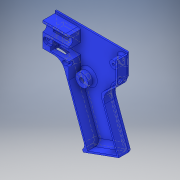
# Autodesk Inventor part: Griff_rechts
Saved by Autodesk Inventor 2019 (Build 230136000, 136)
## iProperties
Created: 2021-03-07
Part Number: Griff_rechts
Material: Generic
Document SubType Name: Modeling
Designer: Lukas
Density: 1 g/cm^3
Appearance: Default
Author: Lukas
Autodesk Inventor part; units mm, degrees
ref_plane "YZ Plane" through (0, 0, 0) normal (1, 0, 0) x (0, 1, 0)
ref_plane "XZ Plane" through (0, 0, 0) normal (0, 1, 0) x (-1, 0, 0)
ref_plane "XY Plane" through (0, 0, 0) normal (0, 0, 1) x (1, 0, 0)
sketch "Sketch1" plane through (0, 0, 0) normal (0, 0, 1) x (1, 0, 0)
  line L0 (-51.5891, 42.2862) -> (-20.8072, -42.2862)
  line L1 (-20.8072, -42.2862) -> (-24.5184, -46.7089)
  line L2 (-24.5184, -46.7089) -> (-23.4923, -49.528)
  line L3 (-23.4923, -49.528) -> (23.4923, -32.427)
  line L4 (21.261, 47.2862) -> (1.261, 28.653)
  line L5 (1.261, 28.653) -> (23.4923, -32.427)
  line L6 (0, -74.8908) -> (0, 102.649) projected
  line L7 (-76.5891, 77.2862) -> (21.261, 77.2862)
  line L8 (21.261, 77.2862) -> (21.261, 47.2862)
  line L9 (-51.5891, 42.2862) -> (-76.5891, 42.2862)
  line L10 (-76.5891, 42.2862) -> (-76.5891, 77.2862)
  point P0 (0, 0)
  point P1 (-36.1981, 0)
  point P2 (0, -40.9775)
  dimension "d1" = 90
  dimension "d2" = 120
  dimension "d3" = 3
  dimension "d5" = 45
  dimension "d6" = 20
  dimension "d7" = 65
  dimension "d8" = 5
  dimension "d10" = 30
  dimension "d30" = 20
  dimension "d31" = 25
  dimension "d32" = 35
  constraints: 21 end point, 5 perpendicular, 2 midpoint, 1 horizontal, 1 horizontal alignment, 1 parallel, 1 vertical alignment
  measures "d1" distance of L0.start L0.end
  measures "d2" angle of L0 L1
  measures "d3" distance of L1.end L2.end
  measures "d5" distance between parallel lines of L5 L0
  measures "d6" angle of L6 L0
  measures "d7" distance of L4.end L3.end
  measures "d8" distance between parallel lines of L2 L0
  measures "d10" distance of L7.end L4.start
  measures "d30" distance from line of L8 L4.end
  measures "d31" distance of L0.start L9.end
  measures "d32" distance of L9.end L7.start
extrude "Extrusion1" add sketch "Sketch1" along normal blind 2
sketch "Sketch2" plane through (0, 0, 2) normal (0, 0, 1) x (1, 0, 0)
  line L0 (-51.5891, 42.2862) -> (-20.8072, -42.2862) projected
  line L1 (-20.8072, -42.2862) -> (-24.5184, -46.7089) projected
  line L2 (-24.5184, -46.7089) -> (-23.4923, -49.528) projected
  line L3 (-23.4923, -49.528) -> (23.4923, -32.427) projected
  line L4 (23.4923, -32.427) -> (1.261, 28.653) projected
  line L5 (1.261, 28.653) -> (21.261, 47.2862) projected
  line L6 (21.261, 47.2862) -> (21.261, 77.2862) projected
  line L7 (21.261, 77.2862) -> (-76.5891, 77.2862) projected
  circle A0 centre (-32.3938, 24.6332) radius 3
  circle A1 centre (-32.3938, 24.6332) radius 8.5
  line L8 (-76.5891, 77.2862) -> (-76.5891, 42.2862) projected
  line L9 (-76.5891, 42.2862) -> (-51.5891, 42.2862) projected
  point P0 (0, 0)
  dimension "d14" = 20
  dimension "d15" = 33
  dimension "d55" = 6
  dimension "d56" = 17
  constraints: 2 centre point, 1 coincident
  measures "d14" distance from line of L5 A0.centre
  measures "d15" distance from line of L4 A0.centre
  measures "d55" diameter of A0
  measures "d56" diameter of A1
extrude "Extrusion2" add sketch "Sketch2" along normal blind 9 contours A1
sketch "Sketch3" plane through (0, 0, 2) normal (0, 0, 1) x (1, 0, 0)
  line L0 (-51.5891, 42.2862) -> (-20.8072, -42.2862) projected
  line L1 (-20.8072, -42.2862) -> (-24.5184, -46.7089) projected
  line L2 (-24.5184, -46.7089) -> (-23.4923, -49.528) projected
  line L3 (-23.4923, -49.528) -> (23.4923, -32.427) projected
  line L4 (23.4923, -32.427) -> (1.261, 28.653) projected
  line L5 (1.261, 28.653) -> (21.261, 47.2862) projected
  line L6 (21.261, 47.2862) -> (21.261, 77.2862) projected
  line L7 (21.261, 77.2862) -> (-76.5891, 77.2862) projected
  circle A0 centre (-32.3938, 24.6332) radius 8.5 projected
  line L8 (-50.1886, 44.2862) -> (-17.5985, -45.2545)
  line L9 (-17.5985, -45.2545) -> (20.9289, -31.2317)
  line L10 (20.9289, -31.2317) -> (-1.0714, 29.2135)
  line L11 (-1.0714, 29.2135) -> (19.261, 48.1563)
  line L12 (19.261, 48.1563) -> (19.261, 77.2862)
  line L13 (21.261, 77.2862) -> (-76.5891, 77.2862) projected
  line L14 (1.261, 28.653) -> (21.261, 47.2862) projected
  line L15 (23.4923, -32.427) -> (1.261, 28.653) projected
  line L16 (-51.5891, 42.2862) -> (-20.8072, -42.2862) projected
  line L17 (-24.5184, -46.7089) -> (-20.8072, -42.2862) projected
  line L18 (-51.5891, 42.2862) -> (-20.8072, -42.2862)
  line L19 (-20.8072, -42.2862) -> (-24.5184, -46.7089)
  line L20 (-24.5184, -46.7089) -> (-23.4923, -49.528)
  line L21 (23.4923, -32.427) -> (-23.4923, -49.528)
  line L22 (-23.4923, -49.528) -> (23.4923, -32.427) projected
  line L23 (23.4923, -32.427) -> (1.261, 28.653)
  line L24 (1.261, 28.653) -> (21.261, 47.2862)
  line L25 (21.261, 77.2862) -> (21.261, 47.2862)
  line L26 (19.261, 77.2862) -> (21.261, 77.2862)
  line L27 (-76.5891, 77.2862) -> (-76.5891, 42.2862) projected
  line L28 (-76.5891, 42.2862) -> (-51.5891, 42.2862) projected
  line L29 (-76.5891, 77.2862) -> (-76.5891, 42.2862) projected
  line L30 (-51.5891, 42.2862) -> (-76.5891, 42.2862)
  line L31 (-76.5891, 42.2862) -> (-76.5891, 44.2862)
  line L32 (-76.5891, 44.2862) -> (-50.1886, 44.2862)
  point P0 (-51.5891, 77.2862)
  dimension "d20" = 2
  dimension "d21" = 2
  dimension "d22" = 2
  dimension "d23" = 2
  dimension "d24" = 2
  dimension "d33" = 2
  constraints: 32 end point, 6 perpendicular, 5 parallel, 2 point on line, 2 vertical, 1 collinear, 1 horizontal
  measures "d20" distance between parallel lines of L6 L12
  measures "d21" distance between parallel lines of L16 L8
  measures "d22" distance between parallel lines of L4 L10
  measures "d23" distance between parallel lines of L14 L11
  measures "d24" distance between parallel lines of L3 L9
  measures "d33" distance between parallel lines of L32 L28
extrude "Extrusion3" add sketch "Sketch3" along normal blind 16 contours L28 L27 L32 L8 L9 L10 L11 L12 L7 L6 L5 L4 L3 L2 L1 L0
fillet "Fillet1" radius 6 2 edges at (9.9288, -1.0091, 2) (1.6652, -38.2431, 2)
fillet "Fillet3" radius 15 2 edges at (1.261, 28.653, 9) (-51.5891, 42.2862, 9)
fillet "Fillet2" radius 8 3 edges at (21.261, 47.2862, 9) (-20.8072, -42.2862, 9) (-1.0714, 29.2135, 13)
sketch "Sketch4" plane through (0, 0, 2) normal (0, 0, 1) x (1, 0, 0)
  line L0 (-76.5891, 77.2862) -> (-76.5891, 44.2862) projected
  line L1 (-76.5891, 74.2862) -> (-42.3941, 74.2862)
  line L2 (-42.3941, 74.2862) -> (-42.3941, 58.2862)
  line L3 (-42.3941, 58.2862) -> (-76.5891, 58.2862)
  line L4 (-76.5891, 58.2862) -> (-76.5891, 74.2862)
  line L5 (19.261, 77.2862) -> (-76.5891, 77.2862) projected
  line L6 (-50.1886, 44.2862) -> (-76.5891, 44.2862) projected
  point P0 (0, 0)
  point P1 (11.261, 77.2862)
  point P2 (-76.5891, 52.2862)
  point P3 (-59.2913, 46.2862)
  dimension "d34" = 34.195
  dimension "d35" = 3
  dimension "d42" = 14
  constraints: 8 end point, 2 parallel, 1 horizontal, 1 perpendicular, 1 point on line, 1 other
  measures "d34" distance of L1.start L1.end
  measures "d35" distance between parallel lines of L5 L1
extrude "Extrusion4" add sketch "Sketch4" along normal blind 16
sketch "Sketch5" plane through (-76.5891, 77.2862, 0) normal (-1, 0, 0) x (0, 0, 1)
  line L0 (18, -3) -> (18, -19) projected
  circle A0 centre (18, -11) radius 5
  point P0 (0, -77.2862)
  dimension "d39" = 10
  constraints: 1 centre point, 1 midpoint
  measures "d39" diameter of A0
extrude "Extrusion5" cut sketch "Sketch5" against normal up to surface (34.195 mm away)
sketch "Sketch6" plane through (0, 0, 2) normal (0, 0, 1) x (1, 0, 0)
  line L0 (-42.3941, 58.2862) -> (-76.5891, 58.2862) projected
  line L1 (-76.5891, 58.2862) -> (-76.5891, 44.2862)
  line L2 (-66.5891, 44.2862) -> (-66.5891, 58.2862)
  line L3 (-76.5891, 58.2862) -> (-66.5891, 58.2862)
  line L4 (-66.5891, 44.2862) -> (-76.5891, 44.2862)
  point P0 (0, 0)
  dimension "d53" = 10
  constraints: 8 end point, 1 coincident, 1 collinear, 1 horizontal, 1 parallel, 1 perpendicular
  measures "d53" distance between parallel lines of L1 L2
extrude "Extrusion6" add sketch "Sketch6" along normal blind 16
sketch "Sketch7" plane through (0, 0, 18) normal (0, 0, 1) x (1, 0, 0)
  circle A0 centre (-72.0891, 53.2862) radius 4
  circle A1 centre (-72.0891, 53.2862) radius 1.45
  line L0 (-72.0891, 57.2862) -> (-66.5891, 57.2862)
  line L1 (-72.0891, 49.2862) -> (-66.5891, 49.2862)
  line L2 (-66.5891, 44.2862) -> (-66.5891, 58.2862) projected
  line L3 (-66.5891, 58.2862) -> (-42.3941, 58.2862) projected
  point P0 (0, 0)
  point P1 (-66.5891, 51.2862)
  dimension "d47" = 2.9
  dimension "d48" = 8
  dimension "d54" = 5.5
  dimension "d66" = 5
  constraints: 4 end point, 2 centre point, 2 horizontal, 2 point on circle, 2 point on line, 2 tangent, 1 coincident, 1 midpoint
  measures "d47" diameter of A1
  measures "d48" diameter of A0
  measures "d54" distance from line of L2 A0.centre
  measures "d66" distance from line of A0.centre L3
extrude "Extrusion7" cut sketch "Sketch7" against normal blind 3
extrude "Extrusion8" cut sketch "Sketch7" against normal blind 15 contours A1
sketch "Sketch8" plane through (0, 0, 2) normal (0, 0, 1) x (1, 0, 0)
  line L0 (-22.387, -37.9459) -> (-51.5891, 42.2862) projected
  line L1 (-17.5985, -45.2545) -> (-50.1886, 44.2862) projected
  line L2 (-76.5891, 42.2862) -> (-62.0922, 42.2862) projected
  line L3 (-50.1886, 44.2862) -> (-66.5891, 44.2862) projected
  line L4 (-42.3941, 58.2862) -> (-66.5891, 58.2862) projected
  line L5 (-66.5891, 58.2862) -> (-42.3941, 58.2862) projected
  line L6 (-42.3941, 71.2862) -> (-42.3941, 61.2862) projected
  line L7 (-42.3941, 71.2862) -> (-42.3941, 74.2862) projected
  line L8 (-42.3941, 74.2862) -> (-42.3941, 58.2862) projected
  circle A0 centre (-32.3938, 24.6332) radius 8.5 projected
  circle A1 centre (-32.3938, 24.6332) radius 8.5 projected
  line L9 (-50.1886, 44.2862) -> (-42.3941, 44.2862)
  line L10 (-42.3941, 44.2862) -> (-42.3941, 22.8707)
  line L11 (-42.3941, 22.8707) -> (-50.1886, 44.2862)
  line L12 (-42.3941, 58.2862) -> (-42.3941, 61.2862) projected
  line L13 (-66.5891, 44.2862) -> (-50.1886, 44.2862) projected
  line L14 (-17.5985, -45.2545) -> (-19.6506, -39.6163) projected
  line L15 (-50.1886, 44.2862) -> (-19.6506, -39.6163) projected
  line L16 (-66.5891, 44.2862) -> (-50.1886, 44.2862) projected
  line L17 (-62.0922, 42.2862) -> (-76.5891, 42.2862) projected
  point P0 (0, 0)
  point P1 (-48.7882, 46.2862)
  point P2 (-48.7882, 46.2862)
  point P3 (-48.7882, 46.2862)
  constraints: 6 end point, 2 collinear, 2 horizontal, 1 perpendicular, 1 point on line, 1 other
extrude "Extrusion9" add sketch "Sketch8" along normal blind 16 contours L1 L9 L10
sketch "Sketch9" plane through (0, 0, 18) normal (0, 0, 1) x (1, 0, 0)
  circle A0 centre (-47.6301, 40.2862) radius 3
  line L0 (-45.3941, 42.2862) -> (-42.3941, 42.2862)
  line L1 (-42.3941, 44.2862) -> (-42.3941, 22.8707) projected
  line L2 (-45.3941, 38.2862) -> (-42.3941, 38.2862)
  line L3 (-42.3941, 22.8707) -> (-42.3941, 44.2862) projected
  line L4 (-42.3941, 44.2862) -> (-66.5891, 44.2862) projected
  point P0 (0, 0)
  point P1 (-66.5891, 44.2862)
  point P2 (-59.2913, 46.2862)
  dimension "d60" = 6
  dimension "d61" = 4
  dimension "d62" = 3
  dimension "d63" = 4
  constraints: 4 end point, 2 point on circle, 2 point on line, 1 centre point, 1 horizontal, 1 perpendicular, 1 vertical alignment, 1 other
  measures "d60" diameter of A0
  measures "d61" distance between parallel lines of L2 L0
  measures "d62" distance of L0.start L0.end
extrude "Extrusion10" cut sketch "Sketch9" against normal blind 5
sketch "Sketch10" plane through (0, 0, 18) normal (0, 0, 1) x (1, 0, 0)
  line L0 (-76.5891, 71.2862) -> (-42.3941, 71.2862) projected
  line L1 (-42.3941, 61.2862) -> (-76.5891, 61.2862) projected
  line L2 (-76.5891, 61.2862) -> (-76.5891, 71.2862) projected
  line L3 (-76.5891, 74.2862) -> (-76.5891, 71.2862) projected
  line L4 (-76.5891, 77.2862) -> (-76.5891, 74.2862) projected
  line L5 (-76.5891, 42.2862) -> (-76.5891, 77.2862) projected
  line L6 (-76.5891, 61.2862) -> (-76.5891, 42.2862) projected
  line L7 (-42.3941, 71.2862) -> (-42.3941, 61.2862) projected
  line L8 (-42.3941, 58.2862) -> (-42.3941, 61.2862) projected
  line L9 (-42.3941, 74.2862) -> (-42.3941, 58.2862) projected
  line L10 (-42.3941, 71.2862) -> (-42.3941, 74.2862) projected
  line L11 (-67.3941, 68.5362) -> (-47.3941, 68.5362)
  line L12 (-47.3941, 68.5362) -> (-47.3941, 64.0362)
  line L13 (-47.3941, 64.0362) -> (-67.3941, 64.0362)
  line L14 (-67.3941, 64.0362) -> (-67.3941, 68.5362)
  point P0 (0, 0)
  dimension "d67" = 2.75
  dimension "d68" = 2.75
  dimension "d69" = 4.5
  dimension "d70" = 5
  dimension "d71" = 20
  constraints: 8 end point, 2 parallel, 1 horizontal, 1 perpendicular
  measures "d67" distance between parallel lines of L0 L11
  measures "d68" distance between parallel lines of L1 L13
  measures "d69" distance of L13.end L11.start
  measures "d70" distance between parallel lines of L7 L12
  measures "d71" distance of L11.start L11.end
extrude "Extrusion11" cut sketch "Sketch10" against normal through all contours L11 L12 L13 L14
sketch "Sketch11" plane through (0, 0, 2) normal (0, 0, 1) x (1, 0, 0)
  circle A0 centre (13.261, 67.2862) radius 5
  line L0 (19.261, 77.2862) -> (19.261, 48.1563) projected
  line L1 (19.261, 48.1563) -> (2.8048, 32.8248) projected
  line L2 (8.5288, 35.4241) -> (18.7143, 44.9135) projected
  arc A1 (18.7143, 44.9135) -> (21.261, 50.7669) centre (13.261, 50.7669) ccw projected
  line L3 (21.261, 50.7669) -> (21.261, 77.2862) projected
  line L4 (-76.5891, 77.2862) -> (21.261, 77.2862) projected
  line L5 (19.261, 77.2862) -> (-76.5891, 77.2862) projected
  line L6 (21.261, 77.2862) -> (19.261, 77.2862) projected
  line L7 (0.4724, 33.3853) -> (17.261, 49.0265) projected
  circle A2 centre (13.261, 67.2862) radius 1.45
  line L8 (21.261, 77.2862) -> (21.261, 50.7669) projected
  arc A3 (18.7143, 44.9135) -> (21.261, 50.7669) centre (13.261, 50.7669) ccw projected
  line L9 (18.7143, 44.9135) -> (8.5288, 35.4241) projected
  line L10 (2.8048, 32.8248) -> (1.7313, 31.8246) projected
  line L11 (1.7313, 31.8246) -> (19.261, 48.1563) projected
  line L12 (19.261, 48.1563) -> (19.261, 77.2862) projected
  point P0 (0, 0)
  dimension "d75" = 10
  dimension "d76" = 10
  dimension "d77" = 2.9
  dimension "d121" = 6
  constraints: 2 centre point, 1 coincident
  measures "d75" distance from line of L4 A0.centre
  measures "d76" diameter of A0
  measures "d77" diameter of A2
  measures "d121" distance from line of L0 A0.centre
extrude "Extrusion12" add sketch "Sketch11" along normal blind 13
sketch "Sketch17" plane through (0, 0, 2) normal (0, 0, 1) x (1, 0, 0)
  circle A0 centre (-59.5891, 54.2862) radius 4
  circle A1 centre (-59.5891, 54.2862) radius 1.45
  line L0 (-42.3941, 58.2862) -> (-66.5891, 58.2862) projected
  line L1 (-66.5891, 58.2862) -> (-42.3941, 58.2862) projected
  line L2 (-66.5891, 57.2862) -> (-66.5891, 49.2862) projected
  line L3 (-66.5891, 44.2862) -> (-66.5891, 49.2862) projected
  line L4 (-66.5891, 58.2862) -> (-66.5891, 44.2862) projected
  line L5 (-66.5891, 57.2862) -> (-66.5891, 58.2862) projected
  line L6 (-42.3941, 71.2862) -> (-42.3941, 61.2862) projected
  line L7 (-42.3941, 71.2862) -> (-42.3941, 74.2862) projected
  line L8 (-42.3941, 74.2862) -> (-42.3941, 58.2862) projected
  line L9 (-42.3941, 58.2862) -> (-42.3941, 61.2862) projected
  point P0 (0, 0)
  dimension "d109" = 2.9
  dimension "d110" = 8
  dimension "d111" = 4
  dimension "d112" = 7
  constraints: 2 centre point, 1 coincident
  measures "d109" diameter of A1
  measures "d110" diameter of A0
  measures "d111" distance from line of L0 A0.centre
  measures "d112" distance from line of L2 A0.centre
extrude "Extrusion18" add sketch "Sketch17" along normal blind 3
sketch "Sketch12" plane through (19.261, 48.1563, 18) normal (-1, 0, 0) x (0, 0, 1)
  circle A0 centre (-4, 4) radius 3.5
  line L0 (0, 29.1298) -> (0, 0) projected
  line L1 (-16, 0) -> (0, 0) projected
  point P0 (-18, -48.1563)
  point P1 (-10, 0)
  dimension "d81" = 4
  dimension "d82" = 7
  dimension "d83" = 4
  constraints: 1 centre point
  measures "d81" distance from line of L0 A0.centre
  measures "d82" diameter of A0
  measures "d83" distance from line of L1 A0.centre
extrude "Extrusion13" cut sketch "Sketch12" against normal blind 2
sketch "Sketch14" plane through (-76.5891, 42.2862, 18) normal (0, -1, 0) x (1, 0, 0)
  line L0 (9, -5.8) -> (24, -5.8)
  line L1 (24, -5.8) -> (24, -11)
  line L2 (24, -11) -> (9, -11)
  line L3 (9, -11) -> (9, -5.8)
  line L4 (0, 0) -> (14.4969, 0) projected
  line L5 (0, -18) -> (0, 0) projected
  point P0 (76.5891, -18)
  point P1 (0, -12)
  dimension "d91" = 9
  dimension "d92" = 15
  dimension "d93" = 5.2
  dimension "d122" = 7
  constraints: 8 end point, 2 parallel, 1 perpendicular
  measures "d91" distance between parallel lines of L5 L3
  measures "d92" distance of L1.end L2.end
  measures "d93" distance of L0.end L1.end
  measures "d122" distance from line of L5.start L2
extrude "Extrusion15" cut sketch "Sketch14" against normal blind 4 and the other way blind 4
fillet "Fillet4" radius 3 4 edges at (8.261, 67.2862, 2) (-40.8938, 24.6332, 2) (-2.2369, 23.5656, 2) (10.4961, 39.9905, 2)
chamfer "Chamfer1" distance 1 distance2 4 1 edges at (-42.3941, 74.2862, 10) measured on face at (-42.3941, 73.7862, 10)
chamfer "Chamfer2" distance 1 distance2 4 1 edges at (-67.5891, 46.2862, 9.6) measured on face at (-67.0891, 46.2862, 9.6)
chamfer "Chamfer3" distance 3 angle 60 11 edges at (-35.1919, -2.7647, 0) (-53.4885, 39.5734, 0) (-69.3406, 42.2862, 0) (-22.026, -42.0713, 0) (-24.1473, -46.2667, 0) (14.0753, -6.5541, 0) (4.169, 27.9542, 0) (13.6216, 40.1688, 0) (20.7443, 47.9384, 0) (18.9945, 45.1877, 0) (21.261, 64.0265, 0) measured on face at (-69.3406, 42.7862, 0) measured on face at (13.2807, 40.5347, 0) measured on face at (-23.7642, -46.588, 0) measured on face at (20.2766, 48.1152, 0) measured on face at (-34.722, -2.5937, 0) measured on face at (-21.5336, -42.1581, 0) measured on face at (-53.2017, 39.983, 0) measured on face at (18.6362, 45.5364, 0) measured on face at (13.6055, -6.7251, 0) measured on face at (20.761, 64.0265, 0) measured on face at (3.6829, 28.071, 0)
equation "\"d21\" = d20"
equation "\"d22\" = d20"
equation "\"d23\" = d20"
equation "\"d24\" = d20"
equation "\"d33\" = d20"
equation "\"d68\" = d67"
body "Solid1"
